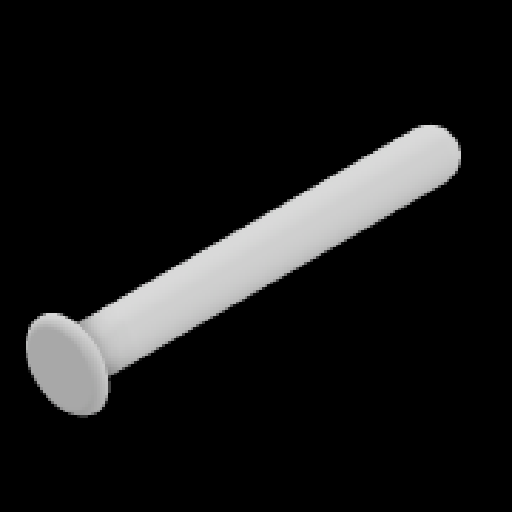
# Autodesk Inventor part: DrivePillars
Saved by Autodesk Inventor 2025 (Build 290162000, 162)
## iProperties
Created: 2024-11-19
Part Number: DrivePillars
Material: Generic
Document SubType Name: Modeling
Designer: Trevor
Density: 1 g/cm^3
Appearance: Default
Author: Trevor
Autodesk Inventor part; units mm, degrees
ref_plane "YZ Plane" through (0, 0, 0) normal (1, 0, 0) x (0, 1, 0)
ref_plane "XZ Plane" through (0, 0, 0) normal (0, 1, 0) x (-1, 0, 0)
ref_plane "XY Plane" through (0, 0, 0) normal (0, 0, 1) x (1, 0, 0)
sketch "Sketch1" plane through (0, 0, 0) normal (0, 0, 1) x (1, 0, 0)
  circle A0 centre (108.5, -103.9) radius 5 projected
  circle A1 centre (108.5, -103.9) radius 9
  point P0 (0, 0)
  dimension "d0" = 4
  constraints: 1 centre point
  measures "d0" radial gap between concentric circles of A0 A1
extrude "Extrusion1" add sketch "Sketch1" along normal blind 2 contours A0 | A1
fillet "Fillet1" radius 2 1 edges at (99.5, -103.9, 2)
sketch "Sketch2" plane through (108.5, -103.9, 0) normal (0, 0, -1) x (-1, 0, 0)
  circle A0 centre (0, 0) radius 5 projected
  point P0 (108.5, 103.9)
extrude "Extrusion3" add sketch "Sketch2" along normal up to surface (86.2427 mm away)
fillet "Fillet2" radius 5 1 edges at (113.5, -103.9, -86.2427)
body "Solid1"
